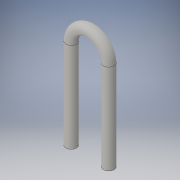
# Autodesk Inventor part: Small_Staple
Saved by Autodesk Inventor 2016 (Build 200138000, 138)
## iProperties
Created: 2017-11-13
Part Number: Small_Staple
Material: Generic
Document SubType Name: Modeling
Designer: shen95841
Density: 1 g/cm^3
Appearance: Default
Author: shen95841
Autodesk Inventor part; units mm, degrees
ref_plane "YZ Plane" through (0, 0, 0) normal (1, 0, 0) x (0, 1, 0)
ref_plane "XZ Plane" through (0, 0, 0) normal (0, 1, 0) x (-1, 0, 0)
ref_plane "XY Plane" through (0, 0, 0) normal (0, 0, 1) x (1, 0, 0)
sketch "Sketch1" plane through (0, 0, 0) normal (0, 0, 1) x (1, 0, 0)
  line L0 (0, 0) -> (0, 11.8618)
  line L1 (4.953, 0) -> (4.953, 11.8618)
  arc A0 (4.953, 11.8618) -> (0, 11.8618) centre (2.4765, 11.8618) ccw
  dimension "d0" = 11.8618
  dimension "d1" = 4.953
  dimension "d2" = 11.8618
  dimension "d3" = 2.4765
  dimension "d4" = 4.953
  constraints: 4 end point, 2 coincident, 2 point on circle, 2 vertical, 1 centre point
  measures "d0" distance of L0.start L0.end
  measures "d1" distance of L1.start L0.start
  measures "d2" distance of L1.start L1.end
  measures "d3" distance of point (2.477, 11.862) L0.end
  measures "d4" distance from line of L1 L0.end
sketch "Sketch2" plane through (0, 0, 0) normal (0, 1, 0) x (-1, 0, 0)
  circle A0 centre (0, 0) radius 0.6985
  dimension "d6" = 1.397
  constraints: 1 centre point, 1 coincident
  measures "d6" diameter of A0
sweep "Sweep1" add profiles "Sketch2" path "Sketch1" path curves L0 A0 L1
body "Solid1"
